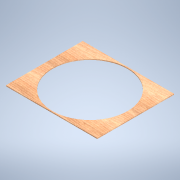
# Autodesk Inventor part: Boden_drehscheibe
Saved by Autodesk Inventor 2021 (Build 250183000, 183)
## iProperties
Created: 2022-06-27
Part Number: Boden_drehscheibe
Material: Holz (Birke)
Document SubType Name: Modeling
Designer: adria
Mass: 223.231 g
Surface Area: 1779.12 cm^2
Volume: 405.875 cm^3
Density: 0.55 g/cm^3
Appearance: Birke - natur - poliert
Author: adria
Autodesk Inventor part; units mm, degrees
ref_plane "YZ Plane" through (0, 0, 0) normal (1, 0, 0) x (0, 1, 0)
ref_plane "XZ Plane" through (0, 0, 0) normal (0, 1, 0) x (-1, 0, 0)
ref_plane "XY Plane" through (0, 0, 0) normal (0, 0, 1) x (1, 0, 0)
sketch "Skizze1" plane through (0, 0, 0) normal (0, 1, 0) x (-1, 0, 0)
  line L0 (-250, 210) -> (250, 210)
  line L1 (250, 210) -> (250, -210)
  line L2 (250, -210) -> (-250, -210)
  line L3 (-250, -210) -> (-250, 210)
  line L4 (-250, 210) -> (250, -210) construction
  line L5 (250, 210) -> (-250, -210) construction
  circle A0 centre (0, 0) radius 202.5
  dimension "d0" = 500
  dimension "d1" = 420
  dimension "d2" = 405
  constraints: 12 end point, 2 midpoint, 2 parallel, 1 centre point, 1 coincident, 1 horizontal, 1 perpendicular
  measures "d0" distance of L1.end L2.end
  measures "d1" distance of L0.end L1.end
  measures "d2" diameter of A0
extrude "Extrusion1" add sketch "Skizze1" along normal blind 5
